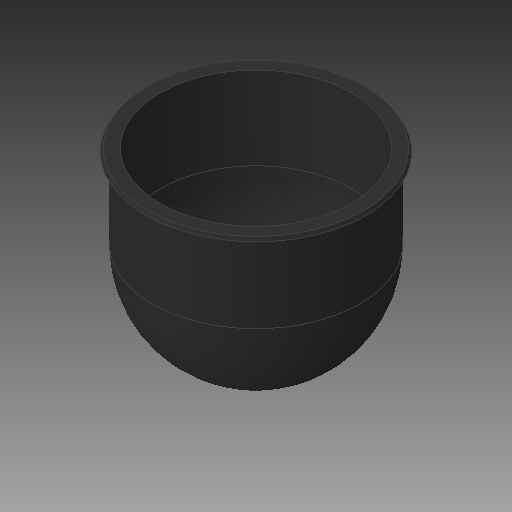
# Autodesk Inventor part: PivotCup
Saved by Autodesk Inventor 2019 (Build 230136000, 136)
## iProperties
Created: 2020-12-10
Part Number: PivotCup
Material: Rubber, Black
Document SubType Name: Modeling
Designer: Anass Hamdi
Density: 0.93 g/cm^3
Appearance: Rubber - Black
Author: Anass Hamdi
Autodesk Inventor part; units mm, degrees
ref_plane "YZ Plane" through (0, 0, 0) normal (1, 0, 0) x (0, 1, 0)
ref_plane "XZ Plane" through (0, 0, 0) normal (0, 1, 0) x (-1, 0, 0)
ref_plane "XY Plane" through (0, 0, 0) normal (0, 0, 1) x (1, 0, 0)
sketch "Sketch1" plane through (0, 0, 0) normal (0, 0, 1) x (1, 0, 0)
  line L0 (-6, 0) -> (-6, -5)
  arc A0 (-6, -5) -> (0, -11) centre (0, -5) ccw
  line L1 (0, -11) -> (0, -11.5)
  line L2 (-6.5, 0) -> (-6.5, -5)
  line L3 (-6, 0) -> (-6, 0.2)
  line L4 (-6.5, 0) -> (-6.9, 0)
  line L5 (-6.7654, 0.2) -> (-6, 0.2)
  line L6 (-6.9, 0) -> (-6.7654, 0.2)
  arc A1 (-6.5, -5) -> (0, -11.5) centre (0, -5) ccw
  point P0 (0, -11.5)
  dimension "d3" = 0.5
  dimension "d5" = 0.2
  dimension "d6" = 0.4
  dimension "d8" = 0.5
  constraints: 14 end point, 4 point on circle, 4 vertical, 2 centre point, 1 coincident, 1 horizontal
  measures "d3" distance of L1.end L1.start
  measures "d5" distance of L0.start L3.end
  measures "d6" distance of L2.start L4.end
  measures "d8" distance between parallel lines of L0 L2
revolve "Revolution1" add sketch "Sketch1" angle 360 about axis through (0, -11, 0) along (0, -1, 0)
body "Solid1"
